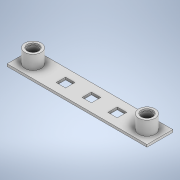
# Autodesk Inventor part: VexLegoMount
Saved by Autodesk Inventor 2020 (Build 240168000, 168)
## iProperties
Created: 2020-02-28
Part Number: VexLegoMount
Material: Generic
Document SubType Name: Modeling
Designer: Luke
Density: 1 g/cm^3
Appearance: Default
Author: Luke
Autodesk Inventor part; units mm, degrees
ref_plane "YZ Plane" through (0, 0, 0) normal (1, 0, 0) x (0, 1, 0)
ref_plane "XZ Plane" through (0, 0, 0) normal (0, 1, 0) x (-1, 0, 0)
ref_plane "XY Plane" through (0, 0, 0) normal (0, 0, 1) x (1, 0, 0)
sketch "Sketch1" plane through (0, 0, 0) normal (0, 1, 0) x (-1, 0, 0)
  line L0 (22.352, 6.35) -> (-46.355, 6.35)
  line L1 (-46.355, 6.35) -> (-46.355, -6.35)
  line L2 (-46.355, -6.35) -> (22.352, -6.35)
  line L3 (22.352, -6.35) -> (22.352, 6.35)
  line L4 (-2.3114, -2.3114) -> (2.3114, -2.3114)
  line L5 (2.3114, -2.3114) -> (2.3114, 2.3114)
  line L6 (2.3114, 2.3114) -> (-2.3114, 2.3114)
  line L7 (-2.3114, 2.3114) -> (-2.3114, -2.3114)
  line L8 (-2.3114, -2.3114) -> (2.3114, 2.3114) construction
  line L9 (2.3114, -2.3114) -> (-2.3114, 2.3114) construction
  line L10 (-10.3886, 2.3114) -> (-15.0114, 2.3114)
  line L11 (-15.0114, 2.3114) -> (-15.0114, -2.3114)
  line L12 (-15.0114, -2.3114) -> (-10.3886, -2.3114)
  line L13 (-10.3886, -2.3114) -> (-10.3886, 2.3114)
  line L14 (-10.3886, 2.3114) -> (-15.0114, -2.3114) construction
  line L15 (-15.0114, 2.3114) -> (-10.3886, -2.3114) construction
  line L16 (-23.0886, 2.3114) -> (-27.7114, 2.3114)
  line L17 (-27.7114, 2.3114) -> (-27.7114, -2.3114)
  line L18 (-27.7114, -2.3114) -> (-23.0886, -2.3114)
  line L19 (-23.0886, -2.3114) -> (-23.0886, 2.3114)
  line L20 (-23.0886, 2.3114) -> (-27.7114, -2.3114) construction
  line L21 (-27.7114, 2.3114) -> (-23.0886, -2.3114) construction
  point P0 (0, 0)
  point P1 (-12.7, 0)
  point P2 (-25.4, 0)
  dimension "d0" = 68.707
  dimension "d1" = 12.7
  dimension "d2" = 4.6228
  dimension "d3" = 4.6228
  dimension "d4" = 4.6228
  dimension "d5" = 4.6228
  dimension "d6" = 12.7
  dimension "d7" = 12.7
  dimension "d8" = 6.35
  dimension "d9" = 22.352
  constraints: 44 end point, 8 parallel, 6 midpoint, 4 horizontal, 4 perpendicular, 1 point on line
  measures "d0" distance of L2.end L1.end
  measures "d1" distance of L1.end L0.end
  measures "d2" distance of L6.end L5.end
  measures "d3" distance of L5.end L4.end
  measures "d4" distance of L12.end L11.end
  measures "d5" distance of L18.end L17.end
  measures "d6" distance of point (-12.7, 0) point (0, 0)
  measures "d7" distance of point (-25.4, 0) point (-12.7, 0)
  measures "d8" distance from line of L2 point (0, 0)
  measures "d9" distance from line of L3 point (0, 0)
extrude "Extrusion1" add sketch "Sketch1" along normal blind 1.1684
sketch "Sketch2" plane through (0, 1.1684, 0) normal (0, 1, 0) x (1, 0, 0)
  line L0 (-22.352, 6.35) -> (-22.352, -6.35) projected
  circle A0 centre (-16.002, 0) radius 4.0259
  point P0 (0, 0)
  dimension "d12" = 6.35
  dimension "d13" = 8.0518
  constraints: 1 centre point, 1 coincident
  measures "d12" distance from line of L0 point (-16.002, 0)
  measures "d13" diameter of A0
extrude "Extrusion2" add sketch "Sketch2" along normal blind 6.8326
sketch "Sketch3" plane through (-16.002, 8.001, 0) normal (0, 1, 0) x (1, 0, 0)
  circle A0 centre (0, 0) radius 2.8575
  point P0 (16.002, 0)
  dimension "d16" = 5.715
  constraints: 1 centre point
  measures "d16" diameter of A0
extrude "Extrusion3" cut sketch "Sketch3" against normal blind 0.7874
sketch "Sketch4" plane through (0, 0, 0) normal (0, -1, 0) x (1, 0, 0)
  circle A0 centre (-16.002, 0) radius 2.8575 projected
  circle A1 centre (-16.002, 0) radius 2.8575
  point P0 (0, 0)
  constraints: 1 centre point, 1 coincident
extrude "Extrusion4" cut sketch "Sketch4" against normal blind 0.7874
sketch "Sketch5" plane through (-16.002, 7.2136, 0) normal (0, 1, 0) x (1, 0, 0)
  circle A0 centre (0, 0) radius 2.4511
  point P0 (16.002, 0)
  dimension "d21" = 4.9022
  constraints: 1 centre point
  measures "d21" diameter of A0
extrude "Extrusion5" cut sketch "Sketch5" against normal through all
sketch "Sketch6" plane through (0, 1.1684, 0) normal (0, 1, 0) x (1, 0, 0)
  line L0 (46.355, -6.35) -> (46.355, 6.35) projected
  circle A0 centre (40.005, 0) radius 4.0259
  point P0 (0, 0)
  dimension "d24" = 6.35
  dimension "d25" = 8.0518
  constraints: 1 centre point, 1 coincident
  measures "d24" distance from line of point (40.005, 0) L0
  measures "d25" diameter of A0
extrude "Extrusion6" add sketch "Sketch6" along normal blind 6.8326
sketch "Sketch7" plane through (40.005, 8.001, 0) normal (0, 1, 0) x (1, 0, 0)
  circle A0 centre (0, 0) radius 2.8575
  point P0 (-40.005, 0)
  dimension "d28" = 5.715
  constraints: 1 centre point
  measures "d28" diameter of A0
extrude "Extrusion7" cut sketch "Sketch7" against normal blind 0.7874
sketch "Sketch8" plane through (0, 0, 0) normal (0, -1, 0) x (1, 0, 0)
  circle A0 centre (40.005, 0) radius 2.8575 projected
  circle A1 centre (40.005, 0) radius 2.8575
  point P0 (0, 0)
  constraints: 1 centre point, 1 coincident
extrude "Extrusion8" cut sketch "Sketch8" against normal blind 0.7874
sketch "Sketch9" plane through (40.005, 7.2136, 0) normal (0, 1, 0) x (1, 0, 0)
  circle A0 centre (0, 0) radius 2.4511
  point P0 (-40.005, 0)
  dimension "d33" = 4.9022
  constraints: 1 centre point
  measures "d33" diameter of A0
extrude "Extrusion9" cut sketch "Sketch9" against normal through all
body "Solid1"
